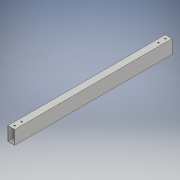
# Autodesk Inventor part: 1x2 28in
Saved by Autodesk Inventor 2018 (Build 220112000, 112)
## iProperties
Created: 2019-01-11
Part Number: 1x2 28in
Material: Generic
Document SubType Name: Modeling
Designer: s-2512711
Density: 1 g/cm^3
Appearance: Default
Author: s-2512711
Autodesk Inventor part; units mm, degrees
ref_plane "YZ Plane" through (0, 0, 0) normal (1, 0, 0) x (0, 1, 0)
ref_plane "XZ Plane" through (0, 0, 0) normal (0, 1, 0) x (-1, 0, 0)
ref_plane "XY Plane" through (0, 0, 0) normal (0, 0, 1) x (1, 0, 0)
sketch "Sketch1" plane through (0, 0, 0) normal (0, 0, 1) x (1, 0, 0)
  line L0 (0, 0) -> (25.4, 0)
  line L1 (25.4, 0) -> (25.4, 50.8)
  line L2 (25.4, 50.8) -> (0, 50.8)
  line L3 (0, 50.8) -> (0, 0)
  line L4 (23.8125, 1.5875) -> (1.5875, 1.5875)
  line L5 (1.5875, 1.5875) -> (1.5875, 49.2125)
  line L6 (1.5875, 49.2125) -> (23.8125, 49.2125)
  line L7 (23.8125, 49.2125) -> (23.8125, 1.5875)
  dimension "d0" = 25.4
  dimension "d1" = 50.8
  dimension "d2" = 1.5875
  constraints: 16 end point, 4 parallel, 2 perpendicular, 1 horizontal, 3 other
  measures "d0" distance of L2.end L1.end
  measures "d1" distance of L1.end L0.end
  measures "d2" distance between parallel lines of L0 L4
extrude "Extrusion1" add sketch "Sketch1" along normal blind 584.2
sketch "Sketch2" plane through (0, 50.8, 0) normal (0, 1, 0) x (1, 0, 0)
  line L0 (23.8125, 0) -> (1.5875, 0) construction
  line L1 (12.7, 0) -> (12.7, -12.7) construction
  line L2 (25.4, -584.2) -> (0, -584.2) construction
  line L3 (12.7, -584.2) -> (12.7, -571.5) construction
  circle A0 centre (12.7, -571.5) radius 2.5797
  circle A1 centre (12.7, -12.7) radius 2.5797
  point P0 (0, 0)
  dimension "d5" = 12.7
  dimension "d6" = 12.7
  dimension "d7" = 5.1594
  constraints: 4 end point, 2 centre point, 2 coincident, 2 midpoint, 2 vertical
  measures "d5" distance of L1.start L1.end
  measures "d6" distance of L3.start L3.end
  measures "d7" diameter of A0
extrude "Extrusion2" cut sketch "Sketch2" against normal blind 711.2
sketch "Sketch3" plane through (0, 50.8, 0) normal (0, 1, 0) x (1, 0, 0)
  circle A0 centre (12.7, -12.7) radius 2.5797 construction
  line L0 (12.7, -12.7) -> (12.7, -38.1) construction
  circle A1 centre (12.7, -38.1) radius 2.5797
  circle A2 centre (12.7, -571.5) radius 2.5797 construction
  line L1 (12.7, -571.5) -> (12.7, -546.1) construction
  circle A3 centre (12.7, -546.1) radius 2.5797
  point P0 (0, 0)
  dimension "d10" = 25.4
  dimension "d13" = 25.4
  constraints: 4 end point, 2 centre point, 2 coincident, 2 vertical
  measures "d10" distance of L0.start L0.end
  measures "d13" distance of L1.start L1.end
extrude "Extrusion4" cut sketch "Sketch3" against normal blind 68.2625
body "Solid1"
